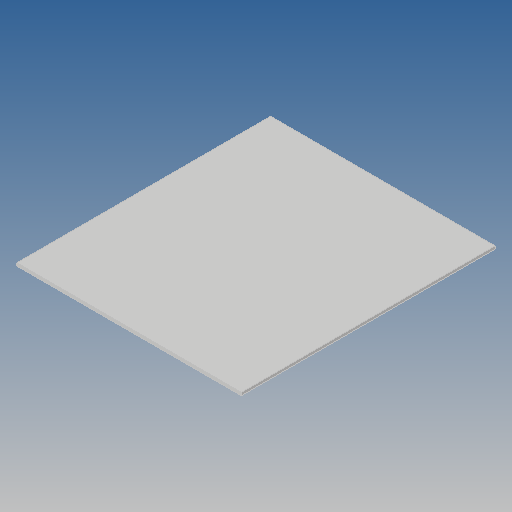
# Autodesk Inventor part: BackPlate
Saved by Autodesk Inventor 2018 (Build 220112000, 112)
## iProperties
Created: 2022-08-30
Part Number: BackPlate
Material: Generic
Document SubType Name: Modeling
Designer: Nathann
Density: 1 g/cm^3
Appearance: Default
Author: Nathann
Autodesk Inventor part; units mm, degrees
ref_plane "YZ Plane" through (0, 0, 0) normal (1, 0, 0) x (0, 1, 0)
ref_plane "XZ Plane" through (0, 0, 0) normal (0, 1, 0) x (-1, 0, 0)
ref_plane "XY Plane" through (0, 0, 0) normal (0, 0, 1) x (1, 0, 0)
sketch "Sketch1" plane through (0, 0, 0) normal (0, 1, 0) x (-1, 0, 0)
  line L0 (-230, -260) -> (230, -260)
  line L1 (230, -260) -> (230, 260)
  line L2 (230, 260) -> (-230, 260)
  line L3 (-230, 260) -> (-230, -260)
  line L4 (-230, -260) -> (230, 260) construction
  line L5 (230, -260) -> (-230, 260) construction
  point P0 (0, 0)
  dimension "d2" = 520
  dimension "d3" = 460
  constraints: 12 end point, 2 midpoint, 2 parallel, 1 horizontal, 1 perpendicular
  measures "d2" distance of L2.end L0.start
  measures "d3" distance of L0.start L0.end
extrude "Extrusion1" add sketch "Sketch1" along normal blind 6
equation "\"d3\" = HorizontalExtrusion"
equation "\"HorizontalExtrusion\" = 460"
equation "\"RodDiameter\" = 8"
equation "\"VerticalBearingOD\" = 16"
equation "\"PrintingClearance\" = 0.2"
equation "\"TubeID\" = 18"
body "Solid1"
